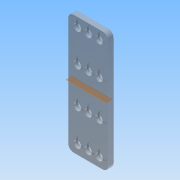
# Autodesk Inventor part: side
Saved by Autodesk Inventor 2015 (Build 190159000, 159)
## iProperties
Created: 2016-01-28
Part Number: side
Material: Plastique PMMA
Document SubType Name: Tôlerie
Designer: Gregwar
Density: 1.188 g/cm^3
Sheet Metal Rule: Par défaut_mm
Appearance: Polycarbonate - Transparent
Author: Gregwar
Autodesk Inventor part; units mm, degrees
ref_plane "YZ Plane" through (0, 0, 0) normal (1, 0, 0) x (0, 1, 0)
ref_plane "XZ Plane" through (0, 0, 0) normal (0, 1, 0) x (-1, 0, 0)
ref_plane "XY Plane" through (0, 0, 0) normal (0, 0, 1) x (1, 0, 0)
sketch "Esquisse1" plane through (0, 0, 0) normal (0, 1, 0) x (-1, 0, 0)
  line L0 (0, 0) -> (22, 0)
  line L1 (22, 0) -> (22, -66)
  line L2 (22, -66) -> (0, -66)
  line L3 (0, -66) -> (0, 0)
  dimension "d0" = 66
  dimension "d1" = 22
  measures "d0" distance of L2.end L0.start
  measures "d1" distance of L0.start L0.end
extrude "Plaque1" add sketch "Esquisse1" along normal blind 3
sketch "Esquisse2" plane through (0, 3, 0) normal (0, 1, 0) x (1, 0, 0)
  line L0 (-22, 0) -> (-22, 66) construction
  line L1 (0, 0) -> (-22, 0) construction
  line L2 (0, 66) -> (0, 0) construction
  line L3 (-22, 66) -> (0, 66) construction
  line L4 (-22, 0) -> (-22, 66) construction
  line L5 (-22, 5) -> (0, 5) construction
  line L6 (0, 66) -> (0, 0) construction
  point P0 (-11, 5)
  point P1 (-17, 5)
  point P2 (-5, 5)
  dimension "d3" = 6
  dimension "d4" = 6
  dimension "d5" = 5
  constraints: 4 point on line, 2 end point, 1 midpoint, 1 perpendicular
  measures "d3" distance of point (-11, 5) point (-17, 5)
  measures "d4" distance of point (-5, 5) point (-11, 5)
  measures "d5" distance between parallel lines of L1 L5
hole "Perçage1" at (-11, 3, -5) at (-17, 3, -5) at (-5, 3, -5) direction (0, -1, 0) diameter 4.05 end through all counterbore diameter 5.5 counterbore depth 1
pattern_linear "Réseau rectangulaire1" count 2 spacing 18 along (0, 0, -1) of "Perçage1"
ref_plane "Plan de construction1" through (-22, 0, -33) normal (0, 0, 1) x (1, 0, 0)
mirror "Symétrie1" about plane through (-22, 0, -33) normal (0, 0, 1) of "Perçage1", "Réseau rectangulaire1"
fillet "Congé1" radius 3 4 edges at (0, 1.5, 0) (0, 1.5, -66) (-22, 1.5, -66) (-22, 1.5, 0)
equation "\"d3\" = ollo_spacing"
equation "\"d4\" = ollo_spacing"
equation "\"d6\" = ollo_hole"
equation "\"d8\" = ollo_ring"
equation "\"d9\" = ollo_depth"
equation "\"d11\" = Epaisseur"
equation "\"d15\" = 3 * ollo_spacing"
equation "\"LargeurGrugeage\" = Epaisseur"
equation "\"ProfondeurGrugeage\" = 0.5 * Epaisseur"
equation "\"TailleGrugeage\" = 4 * Epaisseur"
equation "\"RestesMinimum\" = 2 * Epaisseur"
equation "\"Rayondetransition\" = RayonPli"
equation "\"TailleRayonJacobi\" = RayonPli"
equation "\"TailleJeu\" = Epaisseur"
equation "\"d2\" = RayonPli"
equation "\"ollo_hole\" = 4.05"
equation "\"ollo_ring\" = 5.5"
equation "\"ollo_depth\" = 1"
equation "\"Epaisseur\" = 3"
equation "\"ollo_spacing\" = 6"
equation "\"RayonPli\" = 4"
